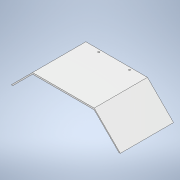
# Autodesk Inventor part: obudowa_górna_dluga
Saved by Autodesk Inventor 2020 (Build 240168000, 168)
## iProperties
Created: 2020-08-31
Part Number: obudowa_górna_dluga
Material: ABS Plastic
Document SubType Name: Modeling
Designer: Hesekiel
Density: 1.06 g/cm^3
Appearance: Smooth - White
Author: Hesekiel
Autodesk Inventor part; units mm, degrees
ref_plane "YZ Plane" through (0, 0, 0) normal (1, 0, 0) x (0, 1, 0)
ref_plane "XZ Plane" through (0, 0, 0) normal (0, 1, 0) x (-1, 0, 0)
ref_plane "XY Plane" through (0, 0, 0) normal (0, 0, 1) x (1, 0, 0)
sketch "Sketch1" plane through (0, 0, 0) normal (0, 0, 1) x (1, 0, 0)
  line L0 (-50, -50) -> (0, 0)
  line L1 (125, 0) -> (0, 0)
  line L2 (125, 0) -> (175, -50)
  line L3 (178, -50) -> (175, -50)
  line L4 (-53, -50) -> (-50, -50)
  circle A0 centre (117.5, -37.5) radius 1.5
  arc A1 (114.25, -43.8002) -> (114.25, -56.1998) centre (117.5, -50) ccw
  arc A2 (120.75, -56.1998) -> (120.75, -43.8002) centre (117.5, -50) ccw
  line L5 (-53, -50) -> (0, 3)
  line L6 (0, 3) -> (125, 3)
  line L7 (125, 3) -> (178, -50)
  constraints: 16 end point, 4 point on circle, 3 centre point, 3 parallel
extrude "Extrusion1" add sketch "Sketch1" along normal blind 108 contours L4 L5 L6 L7 L3 L2 L1 L0
sketch "Sketch2" plane through (0, 3, 0) normal (0, 1, 0) x (1, 0, 0)
  line L0 (0, 0) -> (125, 0)
  line L1 (125, -10) -> (0, -10)
  circle A0 centre (31.25, -5) radius 1.8
  circle A1 centre (93.75, -5) radius 1.8
  line L2 (-53, 32.375) -> (-53, -10)
  line L3 (-53, -10) -> (-50, -10)
  line L4 (-50, -10) -> (0, -10)
  line L5 (0, 0) -> (-53, 0) projected
  line L6 (-53, 0) -> (-53, -108) projected
  line L7 (0, -108) -> (-53, -108) projected
  line L8 (0, 0) -> (0, -108) projected
  circle A2 centre (31.25, -5) radius 1.6
  circle A3 centre (93.75, -5) radius 1.6
  line L9 (125, 0) -> (0, 0) projected
  line L10 (0, 0) -> (0, -108) projected
  line L11 (125, -108) -> (0, -108) projected
  line L12 (125, 0) -> (125, -108) projected
  dimension "d2" = 3.2
  dimension "d3" = 3.2
  constraints: 10 end point, 4 centre point, 2 coincident
  measures "d2" diameter of A2
  measures "d3" diameter of A3
extrude "Extrusion2" cut sketch "Sketch2" against normal up to surface (3 mm away) contours A0 | A1 | A2 | A3
chamfer "Chamfer2" distance 10 angle 45 1 edges at (-51.5, -50, 108)
body "Solid1"
